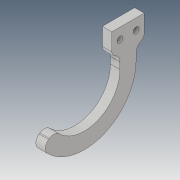
# Autodesk Inventor part: bottomArms2
Saved by Autodesk Inventor 2018 (Build 220112000, 112)
## iProperties
Created: 2020-02-27
Part Number: bottomArms2
Material: Generic
Document SubType Name: Modeling
Designer: anirudh.bali
Density: 1 g/cm^3
Appearance: Default
Author: anirudh.bali
Autodesk Inventor part; units mm, degrees
ref_plane "YZ Plane" through (0, 0, 0) normal (1, 0, 0) x (0, 1, 0)
ref_plane "XZ Plane" through (0, 0, 0) normal (0, 1, 0) x (-1, 0, 0)
ref_plane "XY Plane" through (0, 0, 0) normal (0, 0, 1) x (1, 0, 0)
sketch "Sketch2" plane through (0, 0, 0) normal (1, 0, 0) x (0, 1, 0)
  line L0 (5.3086, -56.9214) -> (-7.3914, -56.9214)
  line L1 (-7.3914, -37.8714) -> (5.3086, -37.8714)
  arc A0 (-33.815, 3.4506) -> (-16.2814, -52.1589) centre (-16.2814, -21.59) ccw
  line L2 (-28.3517, -4.3518) -> (-33.815, 3.4506)
  arc A1 (-28.3517, -4.3518) -> (-16.2814, -42.6339) centre (-16.2814, -21.59) ccw
  line L3 (-4.2164, -37.8714) -> (5.3086, -37.8714)
  line L4 (5.3086, -37.8714) -> (5.3086, -56.9214)
  line L5 (-7.3914, -56.9214) -> (-7.3914, -52.1589)
  line L6 (-7.3914, -42.6339) -> (-7.3914, -37.8714)
  line L7 (-7.3914, -21.59) -> (-7.3914, -42.6339) construction
  line L8 (-7.3914, -52.1589) -> (-7.3914, -56.3416) construction
  line L9 (5.3086, -37.8714) -> (5.3086, -56.9214)
  circle A2 centre (-1.0414, -42.6339) radius 1.75
  circle A3 centre (-1.0414, -42.6339) radius 1.75
  circle A4 centre (-1.0414, -52.1589) radius 1.75
  circle A5 centre (-1.0414, -52.1589) radius 1.75
  line L10 (-7.3914, -42.6339) -> (-16.2814, -42.6339)
  line L11 (-7.3914, -52.1589) -> (-16.2814, -52.1589)
  line L12 (-7.3914, -53.7464) -> (-7.3914, -52.1589)
  line L13 (-7.3914, -42.6339) -> (-7.3914, -41.0464)
  line L14 (-16.2814, -42.6339) -> (-7.3914, -42.6339)
  line L15 (-7.3914, -42.6339) -> (-7.3914, -37.8714)
  line L16 (-7.3914, -37.8714) -> (5.3086, -37.8714)
  line L17 (5.3086, -37.8714) -> (5.3086, -56.9214)
  line L18 (5.3086, -56.9214) -> (-7.3914, -56.9214)
  line L19 (-7.3914, -56.9214) -> (-7.3914, -52.1589)
  line L20 (-7.3914, -52.1589) -> (-16.2814, -52.1589)
  arc A6 (-28.3517, -4.3518) -> (-16.2814, -42.6339) centre (-16.2814, -21.59) ccw
  arc A7 (-33.815, 3.4506) -> (-16.2814, -52.1589) centre (-16.2814, -21.59) ccw
  line L21 (-33.815, 3.4506) -> (-28.3517, -4.3518)
  point P0 (0, 0)
  point P1 (88.5698, 0)
  constraints: 44 end point, 8 centre point, 8 point on circle, 6 collinear, 4 coincident, 3 perpendicular, 1 concentric, 1 parallel
extrude "Extrusion1" add sketch "Sketch2" along normal blind 5.588
fillet "Fillet1" radius 4.445 2 edges at (2.794, -33.815, 3.4506) (2.794, -28.3517, -4.3518)
fillet "Fillet2" radius 5.08 2 edges at (2.794, -7.3914, -42.6339) (2.794, -7.3914, -52.1589)
fillet "Fillet3" radius 3.175 2 edges at (2.794, -7.4013, -37.8714) (2.794, -7.4013, -56.9214)
body "Solid1"
